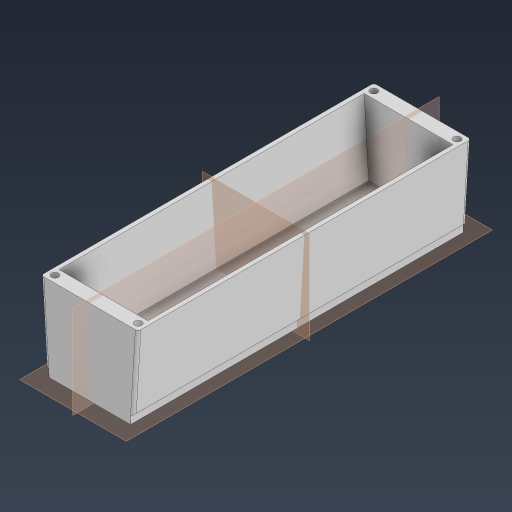
# Autodesk Inventor part: Крепление_новой_колонки
Saved by Autodesk Inventor 2023.2 (Build 272271030, 271C)
## iProperties
Created: 2025-09-17
Part Number: Крепление_новой_колонки
Material: Типовые
Document SubType Name: Modeling
Designer: Олег Коноваленко
Density: 1 g/cm^3
Appearance: По умолчанию
Author: Олег Коноваленко
Autodesk Inventor part; units mm, degrees
sketch "Эскиз4" plane through (0, 0, 0) normal (0, 1, 0) x (-1, 0, 0)
  line L0 (29.5, -120) -> (-29.5, -120)
  line L1 (-29.5, -120) -> (-29.5, 120)
  line L2 (-29.5, 120) -> (29.5, 120)
  line L3 (29.5, 120) -> (29.5, -120)
  line L4 (29.5, -120) -> (-29.5, 120) construction
  line L5 (-29.5, -120) -> (29.5, 120) construction
  point P0 (0, 0)
  dimension "d19" = 59
  dimension "d20" = 240
  constraints: 12 end point, 2 midpoint, 2 parallel, 1 horizontal, 1 perpendicular
  measures "d19" distance of L0.start L0.end
  measures "d20" distance of L0.end L1.end
extrude "Выдавливание4" add sketch "Эскиз4" along normal blind 5
sketch "Эскиз6" plane through (29.5, 0, -120) normal (0, 0, -1) x (-1, 0, 0)
  line L0 (-5.5, 61) -> (64.5, 61)
  line L1 (64.5, 61) -> (61, 5)
  line L2 (61, 5) -> (-2, 5)
  line L3 (-2, 5) -> (-5.5, 61)
  line L4 (29.5, -12) -> (29.5, 72) construction
  line L5 (0, 5) -> (59, 5) projected
  point P0 (29.5, 0)
  point P1 (29.5, 5)
  point P2 (29.5, 5)
  point P3 (29.5, 61)
  dimension "d29" = 63
  dimension "d30" = 70
  dimension "d31" = 56
  constraints: 8 end point, 4 midpoint, 2 point on line, 1 horizontal, 1 parallel
  measures "d29" distance of L1.end L2.end
  measures "d30" distance of L0.start L0.end
  measures "d31" distance between parallel lines of L2 L0
extrude "Выдавливание6" add sketch "Эскиз6" against normal up to surface (240 mm away)
shell "Оболочка5" thickness 3 removed faces 1 at (-11.6667, 61, -40)
sketch "Эскиз7" plane through (-26.5, 3, 117) normal (0, 1, 0) x (1, 0, 0)
  line L0 (0, 0) -> (53, 0) projected
  line L1 (53, 0) -> (53, 234) projected
  line L2 (53, 234) -> (0, 234) projected
  line L3 (0, 234) -> (0, 0) projected
  point P0 (26.5, 117)
extrude "Выдавливание7" add sketch "Эскиз7" along normal blind 5
chamfer "Фаска2" distance 2 angle 45 2 edges at (31.5, 5, 0) (-31.5, 5, 0)
sketch "Эскиз10" plane through (31.9941, 61, 117) normal (0, 0, -1) x (-1, 0, 0)
  line L0 (60.6758, -53) -> (63.9883, 0) projected
  line L1 (3.3125, -53) -> (60.6758, -53) projected
  line L2 (0, 0) -> (3.3125, -53) projected
  line L3 (0, 0) -> (63.9883, 0) projected
  point P0 (31.9941, -61)
extrude "Выдавливание8" add sketch "Эскиз10" along normal blind 7
mirror "Зеркальное отражение1" about plane through (0, 0, 0) normal (0, 0, 1) of "Выдавливание8"
sketch "Эскиз11" plane through (-35, 61, -120) normal (0, 1, 0) x (1, 0, 0)
  circle A0 centre (5, -235) radius 2.55
  circle A1 centre (65, -235) radius 2.55
  circle A2 centre (5, -5) radius 2.55
  circle A3 centre (65, -5) radius 2.55
  line L0 (0, 0) -> (0, -240) projected
  line L1 (0, -5) -> (70, -5) construction
  line L2 (70, 0) -> (70, -240) projected
  line L3 (0, 0) -> (70, 0) projected
  line L4 (0, -235) -> (70, -235) construction
  line L5 (0, -240) -> (70, -240) projected
  point P0 (35, -120)
  dimension "d45" = 5.1
  dimension "d46" = 5
  dimension "d47" = 5
  dimension "d48" = 5
  dimension "d49" = 5
  dimension "d50" = 5
  dimension "d51" = 5
  constraints: 8 point on line, 4 centre point, 4 end point, 3 equal radius, 1 horizontal, 1 perpendicular
  measures "d45" diameter of A2
  measures "d46" distance between parallel lines of L3 L1
  measures "d47" distance between parallel lines of L5 L4
  measures "d48" distance from line of L0 A2.centre
  measures "d49" distance from line of L2 A3.centre
  measures "d50" distance from line of L0 A0.centre
  measures "d51" distance from line of L2 A1.centre
extrude "Выдавливание9" cut sketch "Эскиз11" against normal blind 15 contours A0 | A1 | A2 | A3
sketch "Эскиз12" plane through (0, 0, 0) normal (0, -1, 0) x (1, 0, 0)
  line L0 (15.5, 36.5) -> (-15.5, 36.5) construction
  line L1 (15.5, 42) -> (-15.5, 42)
  line L2 (-15.5, 31) -> (15.5, 31)
  arc A0 (15.5, 31) -> (15.5, 42) centre (15.5, 36.5) ccw
  arc A1 (-15.5, 42) -> (-15.5, 31) centre (-15.5, 36.5) ccw
  line L3 (0, 168) -> (0, -168) projected
  line L4 (-29.5, 120) -> (29.5, 120) projected
  line L5 (-49, 0) -> (49, 0) projected
  point P0 (0, 36.5)
  dimension "d54" = 11
  dimension "d55" = 31
  dimension "d60" = 31
  constraints: 8 end point, 4 point on circle, 4 tangent, 2 centre point, 1 horizontal, 1 midpoint, 1 parallel, 1 point on line
  measures "d54" distance between parallel lines of L1 L2
  measures "d55" distance of L0.end L0.start
  measures "d60" distance between parallel lines of L5 L2
extrude "Выдавливание10" cut sketch "Эскиз12" against normal up to next
fillet "Сопряжение1" radius 2 4 edges at (-33.3124, 33.998, 120) (33.3124, 33.998, 120) (-33.3124, 33.998, -120) (33.3124, 33.998, -120)
sketch "Эскиз13" plane through (-28.6816, 8, 110) normal (0, 1, 0) x (1, 0, 0)
  point P0 (28.6816, 110)
